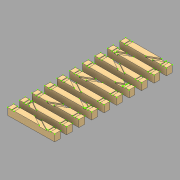
# Autodesk Inventor part: dormentaçãoAmelhor
Saved by Autodesk Inventor 2018 (Build 220112000, 112)
## iProperties
Created: 2019-03-28
Part Number: dormentaçãoAmelhor
Material: Laminated Veneer Lumber
Document SubType Name: Modeling
Designer: Ifes-Vale
Density: 0.51 g/cm^3
Appearance: Plywood - New
Author: Ifes-Vale
Autodesk Inventor part; units mm, degrees
ref_plane "YZ Plane" through (0, 0, 0) normal (1, 0, 0) x (0, 1, 0)
ref_plane "XZ Plane" through (0, 0, 0) normal (0, 1, 0) x (-1, 0, 0)
ref_plane "XY Plane" through (0, 0, 0) normal (0, 0, 1) x (1, 0, 0)
sketch "Sketch2" plane through (0, 0, 0) normal (0, 0, 1) x (1, 0, 0)
  point P0 (264.349385, -5730.127221)
  point P1 (559.859477, -5726.313145)
  point P2 (-178.915755, -5487.873693)
  point P3 (116.594338, -5484.059617)
  point P4 (-663.737, -5225.006632)
  point P5 (-363.609562, -5221.346521)
  point P6 (-677.589036, -4977.200919)
  point P7 (-793.022666, -4978.608654)
  point P8 (-151.211683, -4681.410236)
  point P9 (-451.339121, -4685.099849)
  point P10 (296.670801, -4427.929556)
  point P11 (-3.456637, -4431.61917)
  point P12 (546.007442, -4122.594488)
  point P13 (582.946203, -4121.993825)
  point P14 (144.298409, -3881.152056)
  point P15 (435.191157, -3876.421835)
  point P16 (-372.844253, -3598.273291)
  point P17 (-77.33416, -3595.548009)
  point P18 (-806.874702, -3354.301407)
  point P19 (-525.216644, -3351.703873)
  point P20 (-400.548324, -3051.488745)
  point P21 (-700.675762, -3054.906687)
  point P22 (47.33416, -2798.413483)
  point P23 (-252.793278, -2801.831425)
  point P24 (582.946203, -2497.963106)
  point P25 (287.436111, -2499.067902)
  point P26 (384.40036, -2250.730749)
  point P27 (-141.976993, -1963.360803)
  point P28 (158.150445, -1962.423657)
  point P29 (-594.476822, -1716.799089)
  point P30 (-294.349385, -1715.861943)
  point P31 (-696.058417, -1417.102323)
  point P32 (-252.793278, -1168.024169)
  point P33 (-548.30337, -1168.759844)
  point P34 (264.349385, -877.258052)
  point P35 (-31.160708, -878.112001)
  point P36 (412.104431, -628.856435)
  point P37 (-903.838951, -5745.204739)
  point P38 (-788.405321, -5743.714866)
  point P39 (633.737, -5725.359626)
  point P40 (749.17063, -5723.869752)
  point P41 (-908.456296, -5497.289692)
  point P42 (-793.022666, -5495.799819)
  point P43 (629.119655, -5477.444579)
  point P44 (744.553285, -5475.954706)
  point P45 (-908.456296, -5227.99103)
  point P46 (-793.022666, -5226.583295)
  point P47 (629.119655, -5209.24)
  point P48 (744.553285, -5207.832265)
  point P49 (-913.073641, -4980.072698)
  point P50 (-797.640011, -4978.664963)
  point P51 (629.119655, -4961.265358)
  point P52 (739.93594, -4959.913933)
  point P53 (-913.073641, -4690.776177)
  point P54 (-797.640011, -4689.357095)
  point P55 (624.50231, -4671.874005)
  point P56 (739.93594, -4670.454923)
  point P57 (-917.690986, -4442.858299)
  point P58 (-802.257356, -4441.439217)
  point P59 (624.50231, -4423.899364)
  point P60 (739.93594, -4422.480282)
  point P61 (-917.690986, -4146.395758)
  point P62 (-802.257356, -4144.518686)
  point P63 (624.50231, -4121.318079)
  point P64 (735.318595, -4119.51609)
  point P65 (-917.690986, -3898.421116)
  point P66 (-806.874702, -3896.619127)
  point P67 (619.884965, -3873.41852)
  point P68 (735.318595, -3871.541448)
  point P69 (-922.308332, -3603.340612)
  point P70 (-806.874702, -3602.276049)
  point P71 (619.884965, -3589.118046)
  point P72 (735.318595, -3588.053483)
  point P73 (-922.308332, -3355.365971)
  point P74 (-811.492047, -3354.34399)
  point P75 (615.26762, -3341.185987)
  point P76 (730.70125, -3340.121424)
  point P77 (-926.925677, -3057.483289)
  point P78 (-811.492047, -3056.168696)
  point P79 (615.26762, -3039.920328)
  point P80 (730.70125, -3038.605735)
  point P81 (-926.925677, -2809.508647)
  point P82 (-816.109392, -2808.246638)
  point P83 (615.26762, -2791.945686)
  point P84 (726.083904, -2790.683677)
  point P85 (-931.543022, -2503.62519)
  point P86 (-816.109392, -2503.193628)
  point P87 (610.650274, -2497.859531)
  point P88 (726.083904, -2497.42797)
  point P89 (-931.543022, -2255.650548)
  point P90 (-820.726737, -2255.236249)
  point P91 (610.650274, -2249.884889)
  point P92 (726.083904, -2249.453328)
  point P93 (-936.160367, -1965.840636)
  point P94 (-820.726737, -1965.480195)
  point P95 (610.650274, -1961.010729)
  point P96 (721.466559, -1960.664706)
  point P97 (-936.160367, -1717.865994)
  point P98 (-820.726737, -1717.505553)
  point P99 (606.032929, -1713.050505)
  point P100 (721.466559, -1712.690064)
  point P101 (-940.777712, -1417.711554)
  point P102 (-825.344082, -1417.424181)
  point P103 (606.032929, -1413.860756)
  point P104 (721.466559, -1413.573383)
  point P105 (-940.777712, -1169.736912)
  point P106 (-825.344082, -1169.449539)
  point P107 (601.415584, -1165.897609)
  point P108 (716.849214, -1165.610236)
  point P109 (-945.395058, -880.753908)
  point P110 (-829.961428, -880.420334)
  point P111 (601.415584, -876.284016)
  point P112 (716.849214, -875.950442)
  point P113 (-945.395058, -632.779266)
  point P114 (-829.961428, -632.445692)
  point P115 (601.415584, -628.309374)
  point P116 (712.231869, -627.989143)
  point P117 (-1074.680723, -5747.409752)
  point P118 (915.395058, -5721.724335)
  point P119 (-1074.680723, -5499.43511)
  point P120 (915.395058, -5473.749693)
  point P121 (-1083.915413, -5230.130788)
  point P122 (906.160367, -5205.861436)
  point P123 (-1083.915413, -4982.156146)
  point P124 (906.160367, -4957.886794)
  point P125 (-1088.532759, -4692.933182)
  point P126 (901.543022, -4668.468209)
  point P127 (-1088.532759, -4444.95854)
  point P128 (901.543022, -4420.493567)
  point P129 (-1093.150104, -4149.248907)
  point P130 (896.925677, -4116.888189)
  point P131 (-1093.150104, -3901.274265)
  point P132 (896.925677, -3868.913548)
  point P133 (-1097.767449, -3604.958749)
  point P134 (892.308332, -3586.605677)
  point P135 (-1097.767449, -3356.984107)
  point P136 (892.308332, -3338.631035)
  point P137 (-1107.002139, -3059.534054)
  point P138 (883.073641, -3036.870472)
  point P139 (-1107.002139, -2811.559412)
  point P140 (883.073641, -2788.895831)
  point P141 (-1111.619485, -2504.298425)
  point P142 (878.456296, -2496.858309)
  point P143 (-1111.619485, -2256.323783)
  point P144 (878.456296, -2248.883667)
  point P145 (-1116.23683, -1966.402923)
  point P146 (873.838951, -1960.188924)
  point P147 (-1116.23683, -1718.428282)
  point P148 (873.838951, -1712.214283)
  point P149 (-1125.47152, -1418.171351)
  point P150 (864.60426, -1413.21704)
  point P151 (-1125.47152, -1170.196709)
  point P152 (864.60426, -1165.242399)
  point P153 (-1130.088865, -881.287626)
  point P154 (859.986915, -875.53681)
  point P155 (-1130.088865, -633.312984)
  point P156 (859.986915, -627.562168)
  point P157 (-793.022666, -5042.665596)
  point P158 (-793.022666, -5153.141257)
  point P159 (-793.022666, -5042.665596)
  point P160 (-793.022666, -5153.141257)
  point P161 (619.884965, -4081.420913)
  point P162 (619.884965, -3976.239705)
  point P163 (619.884965, -4081.420913)
  point P164 (619.884965, -3976.239705)
  point P165 (610.650274, -2481.180008)
  point P166 (610.650274, -2315.863581)
  point P167 (610.650274, -2374.7426)
  point P168 (610.650274, -2481.180008)
  point P169 (610.650274, -2315.863581)
  point P170 (610.650274, -2374.7426)
  point P171 (-825.344082, -1325.870433)
  point P172 (-825.344082, -1325.870433)
  point P173 (596.798239, -689.947889)
  point P174 (596.798239, -689.947889)
sketch "Sketch3" plane through (0, 0, 0) normal (0, 0, 1) x (1, 0, 0)
  line L0 (-1130.088865, -633.312984) -> (-1130.088865, -881.287626)
  line L1 (-1130.088865, -881.287626) -> (859.986915, -875.53681)
  line L2 (859.986915, -875.53681) -> (859.986915, -627.562168)
  line L3 (859.986915, -627.562168) -> (-1130.088865, -633.312984)
  line L4 (864.60426, -1165.242399) -> (-1125.47152, -1170.196709)
  line L5 (-1125.47152, -1170.196709) -> (-1125.47152, -1418.171351)
  line L6 (-1125.47152, -1418.171351) -> (864.60426, -1413.21704)
  line L7 (864.60426, -1413.21704) -> (864.60426, -1165.242399)
  line L8 (873.838951, -1712.214283) -> (-1116.23683, -1718.428282)
  line L9 (-1116.23683, -1718.428282) -> (-1116.23683, -1966.402923)
  line L10 (-1116.23683, -1966.402923) -> (873.838951, -1960.188924)
  line L11 (873.838951, -1960.188924) -> (873.838951, -1712.214283)
  line L12 (878.456296, -2248.883667) -> (878.456296, -2496.858309)
  line L13 (878.456296, -2496.858309) -> (-1111.619485, -2504.298425)
  line L14 (-1111.619485, -2504.298425) -> (-1111.619485, -2256.323783)
  line L15 (-1111.619485, -2256.323783) -> (878.456296, -2248.883667)
  line L16 (883.073641, -2788.895831) -> (-1107.002139, -2811.559412)
  line L17 (-1107.002139, -2811.559412) -> (-1107.002139, -3059.534054)
  line L18 (-1107.002139, -3059.534054) -> (883.073641, -3036.870472)
  line L19 (883.073641, -3036.870472) -> (883.073641, -2788.895831)
  line L20 (892.308332, -3338.631035) -> (892.308332, -3586.605677)
  line L21 (892.308332, -3586.605677) -> (-1097.767449, -3604.958749)
  line L22 (-1097.767449, -3604.958749) -> (-1097.767449, -3356.984107)
  line L23 (-1097.767449, -3356.984107) -> (892.308332, -3338.631035)
  line L24 (896.925677, -3868.913548) -> (-1093.150104, -3901.274265)
  line L25 (-1093.150104, -3901.274265) -> (-1093.150104, -4149.248907)
  line L26 (-1093.150104, -4149.248907) -> (896.925677, -4116.888189)
  line L27 (896.925677, -4116.888189) -> (896.925677, -3868.913548)
  line L28 (901.543022, -4420.493567) -> (-1088.532759, -4444.95854)
  line L29 (-1088.532759, -4444.95854) -> (-1088.532759, -4692.933182)
  line L30 (-1088.532759, -4692.933182) -> (901.543022, -4668.468209)
  line L31 (901.543022, -4420.493567) -> (901.543022, -4668.468209)
  line L32 (906.160367, -4957.886794) -> (-1083.915413, -4982.156146)
  line L33 (-1083.915413, -4982.156146) -> (-1083.915413, -5230.130788)
  line L34 (-1083.915413, -5230.130788) -> (906.160367, -5205.861436)
  line L35 (906.160367, -5205.861436) -> (906.160367, -4957.886794)
  line L36 (-1074.680723, -5499.43511) -> (-1074.680723, -5747.409752)
  line L37 (-1074.680723, -5747.409752) -> (915.395058, -5721.724335)
  line L38 (915.395058, -5721.724335) -> (915.395058, -5473.749693)
  line L39 (915.395058, -5473.749693) -> (-1074.680723, -5499.43511)
  point P0 (0, 0)
  constraints: 80 end point, 7 parallel, 6 vertical
extrude "Extrusion1" add sketch "Sketch3" against normal blind 300
sketch "Sketch4" plane through (0, 0, 0) normal (0, 0, 1) x (1, 0, 0)
  line L0 (-903.838951, -5745.204739) -> (-788.405321, -5743.714866)
  line L1 (915.395058, -5721.724335) -> (-1074.680723, -5747.409752)
  line L2 (-793.022666, -5495.799819) -> (-908.456296, -5497.289692)
  line L3 (-908.456296, -5497.289692) -> (-903.838951, -5745.204739)
  line L4 (915.395058, -5473.749693) -> (-1074.680723, -5499.43511)
  line L5 (-788.405321, -5743.714866) -> (-793.022666, -5495.799819)
  line L6 (-793.022666, -5226.583295) -> (-797.640011, -4978.664963)
  line L7 (-797.640011, -4978.664963) -> (-913.073641, -4980.072698)
  line L8 (-1083.915413, -4982.156146) -> (906.160367, -4957.886794)
  line L9 (-908.456296, -5227.99103) -> (-913.073641, -4980.072698)
  line L10 (-793.022666, -5226.583295) -> (-908.456296, -5227.99103)
  line L11 (906.160367, -5205.861436) -> (-1083.915413, -5230.130788)
  line L12 (-797.640011, -4689.357095) -> (-913.073641, -4690.776177)
  line L13 (901.543022, -4668.468209) -> (-1088.532759, -4692.933182)
  line L14 (-913.073641, -4690.776177) -> (-917.690986, -4442.858299)
  line L15 (-917.690986, -4442.858299) -> (-802.257356, -4441.439217)
  line L16 (-1088.532759, -4444.95854) -> (901.543022, -4420.493567)
  line L17 (-802.257356, -4441.439217) -> (-797.640011, -4689.357095)
  line L18 (-917.690986, -4146.395758) -> (-802.257356, -4144.518686)
  line L19 (896.925677, -4116.888189) -> (-1093.150104, -4149.248907)
  line L20 (-802.257356, -4144.518686) -> (-806.874702, -3896.619127)
  line L21 (-806.874702, -3896.619127) -> (-917.690986, -3898.421116)
  line L22 (-1093.150104, -3901.274265) -> (896.925677, -3868.913548)
  line L23 (-917.690986, -4146.395758) -> (-917.690986, -3898.421116)
  line L24 (-922.308332, -3603.340612) -> (-806.874702, -3602.276049)
  line L25 (-806.874702, -3602.276049) -> (-806.874702, -3354.301407)
  line L26 (-806.874702, -3354.301407) -> (-922.308332, -3355.365971)
  line L27 (892.308332, -3338.631035) -> (-1097.767449, -3356.984107)
  line L28 (-922.308332, -3355.365971) -> (-922.308332, -3603.340612)
  line L29 (-926.925677, -3057.483289) -> (-926.925677, -2809.508647)
  line L30 (-926.925677, -2809.508647) -> (-816.109392, -2808.246638)
  line L31 (-1107.002139, -2811.559412) -> (883.073641, -2788.895831)
  line L32 (883.073641, -3036.870472) -> (-1107.002139, -3059.534054)
  line L33 (-811.492047, -3056.168696) -> (-816.109392, -2808.246638)
  line L34 (-926.925677, -3057.483289) -> (-811.492047, -3056.168696)
  line L35 (-931.543022, -2255.650548) -> (-820.726737, -2255.236249)
  line L36 (-1111.619485, -2256.323783) -> (878.456296, -2248.883667)
  line L37 (-816.109392, -2503.193628) -> (-931.543022, -2503.62519)
  line L38 (878.456296, -2496.858309) -> (-1111.619485, -2504.298425)
  line L39 (-931.543022, -2503.62519) -> (-931.543022, -2255.650548)
  line L40 (-820.726737, -2255.236249) -> (-816.109392, -2503.193628)
  line L41 (-820.726737, -1965.480195) -> (-820.726737, -1717.505553)
  line L42 (-820.726737, -1717.505553) -> (-936.160367, -1717.865994)
  line L43 (-1116.23683, -1718.428282) -> (873.838951, -1712.214283)
  line L44 (-820.726737, -1965.480195) -> (-936.160367, -1965.840636)
  line L45 (873.838951, -1960.188924) -> (-1116.23683, -1966.402923)
  line L46 (-936.160367, -1965.840636) -> (-936.160367, -1717.865994)
  line L47 (-825.344082, -1417.424181) -> (-940.777712, -1417.711554)
  line L48 (-940.777712, -1417.711554) -> (-940.777712, -1417.711554)
  line L49 (-940.777712, -1169.736912) -> (-825.344082, -1169.449539)
  line L50 (-825.344082, -1169.449539) -> (-825.344082, -1417.424181)
  line L51 (-940.777712, -1417.711554) -> (-940.777712, -1169.736912)
  line L52 (-945.395058, -880.753908) -> (-945.395058, -632.779266)
  line L53 (-945.395058, -632.779266) -> (-829.961428, -632.445692)
  line L54 (-829.961428, -632.445692) -> (-829.961428, -880.420334)
  line L55 (-829.961428, -880.420334) -> (-829.961428, -880.420334)
  line L56 (-945.395058, -880.753908) -> (-829.961428, -880.420334)
  line L57 (859.986915, -875.53681) -> (-1130.088865, -881.287626)
  point P0 (0, 0)
  constraints: 84 end point, 15 collinear, 3 parallel, 3 vertical
extrude "Extrusion2" cut sketch "Sketch4" against normal blind 25
sketch "Sketch5" plane through (0, 0, 0) normal (0, 0, 1) x (1, 0, 0)
  line L0 (749.17063, -5723.869752) -> (633.737, -5725.359626)
  line L1 (633.737, -5725.359626) -> (629.119655, -5477.444579)
  line L2 (629.119655, -5477.444579) -> (744.553285, -5475.954706)
  line L3 (-1074.680723, -5499.43511) -> (915.395058, -5473.749693)
  line L4 (915.395058, -5721.724335) -> (-1074.680723, -5747.409752)
  line L5 (744.553285, -5475.954706) -> (749.17063, -5723.869752)
  line L6 (744.553285, -5207.832265) -> (629.119655, -5209.24)
  line L7 (906.160367, -5205.861436) -> (-1083.915413, -5230.130788)
  line L8 (629.119655, -5209.24) -> (629.119655, -4961.265358)
  line L9 (629.119655, -4961.265358) -> (739.93594, -4959.913933)
  line L10 (-1083.915413, -4982.156146) -> (906.160367, -4957.886794)
  line L11 (739.93594, -4959.913933) -> (744.553285, -5207.832265)
  line L12 (739.93594, -4670.454923) -> (624.50231, -4671.874005)
  line L13 (624.50231, -4671.874005) -> (624.50231, -4671.874005)
  line L14 (624.50231, -4671.874005) -> (624.50231, -4423.899364)
  line L15 (624.50231, -4423.899364) -> (739.93594, -4422.480282)
  line L16 (739.93594, -4422.480282) -> (739.93594, -4670.454923)
  line L17 (624.50231, -4121.318079) -> (735.318595, -4119.51609)
  line L18 (735.318595, -4119.51609) -> (735.318595, -4119.51609)
  line L19 (735.318595, -4119.51609) -> (735.318595, -3871.541448)
  line L20 (735.318595, -3871.541448) -> (619.884965, -3873.41852)
  line L21 (-1093.150104, -3901.274265) -> (896.925677, -3868.913548)
  line L22 (619.884965, -3873.41852) -> (624.50231, -4121.318079)
  line L23 (619.884965, -3589.118046) -> (735.318595, -3588.053483)
  line L24 (892.308332, -3586.605677) -> (-1097.767449, -3604.958749)
  line L25 (735.318595, -3588.053483) -> (730.70125, -3340.121424)
  line L26 (730.70125, -3340.121424) -> (615.26762, -3341.185987)
  line L27 (-1097.767449, -3356.984107) -> (892.308332, -3338.631035)
  line L28 (615.26762, -3341.185987) -> (619.884965, -3589.118046)
  line L29 (615.26762, -3039.920328) -> (730.70125, -3038.605735)
  line L30 (883.073641, -3036.870472) -> (-1107.002139, -3059.534054)
  line L31 (730.70125, -3038.605735) -> (726.083904, -2790.683677)
  line L32 (615.26762, -2791.945686) -> (726.083904, -2790.683677)
  line L33 (-1107.002139, -2811.559412) -> (883.073641, -2788.895831)
  line L34 (615.26762, -2791.945686) -> (615.26762, -3039.920328)
  line L35 (726.083904, -2497.42797) -> (610.650274, -2497.859531)
  line L36 (610.650274, -2497.859531) -> (610.650274, -2249.884889)
  line L37 (610.650274, -2249.884889) -> (726.083904, -2249.453328)
  line L38 (726.083904, -2249.453328) -> (726.083904, -2249.453328)
  line L39 (878.456296, -2496.858309) -> (-1111.619485, -2504.298425)
  line L40 (726.083904, -2497.42797) -> (726.083904, -2249.453328)
  line L41 (721.466559, -1960.664706) -> (610.650274, -1961.010729)
  line L42 (873.838951, -1960.188924) -> (-820.726737, -1965.480195)
  line L43 (610.650274, -1961.010729) -> (606.032929, -1713.050505)
  line L44 (606.032929, -1713.050505) -> (721.466559, -1712.690064)
  line L45 (-1116.23683, -1718.428282) -> (873.838951, -1712.214283)
  line L46 (721.466559, -1712.690064) -> (721.466559, -1960.664706)
  line L47 (721.466559, -1413.573383) -> (606.032929, -1413.860756)
  line L48 (864.60426, -1413.21704) -> (-825.344082, -1417.424181)
  line L49 (606.032929, -1413.860756) -> (601.415584, -1165.897609)
  line L50 (601.415584, -1165.897609) -> (716.849214, -1165.610236)
  line L51 (-825.344082, -1169.449539) -> (864.60426, -1165.242399)
  line L52 (716.849214, -1165.610236) -> (721.466559, -1413.573383)
  line L53 (601.415584, -628.309374) -> (712.231869, -627.989143)
  line L54 (859.986915, -627.562168) -> (-829.961428, -632.445692)
  line L55 (712.231869, -627.989143) -> (716.849214, -875.950442)
  line L56 (716.849214, -875.950442) -> (601.415584, -876.284016)
  line L57 (-829.961428, -880.420334) -> (859.986915, -875.53681)
  line L58 (601.415584, -876.284016) -> (601.415584, -628.309374)
  point P0 (0, 0)
  constraints: 86 end point, 13 collinear, 4 vertical, 2 parallel
extrude "Extrusion3" cut sketch "Sketch5" against normal blind 25
sketch "Sketch6" plane through (0, 0, 0) normal (0, 0, 1) x (1, 0, 0)
  line L0 (601.415584, -876.284016) -> (601.415584, -628.309374)
  line L1 (-825.344082, -1169.449539) -> (-825.344082, -1417.424181)
  line L2 (610.650274, -2497.859531) -> (610.650274, -2249.884889)
  line L3 (624.50231, -4121.318079) -> (619.884965, -3873.41852)
  line L4 (-797.640011, -4978.664963) -> (-793.022666, -5226.583295)
  line L5 (559.859477, -5726.313145) -> (116.594338, -5484.059617)
  line L6 (116.594338, -5484.059617) -> (-178.915755, -5487.873693)
  line L7 (629.119655, -5477.444579) -> (-793.022666, -5495.799819)
  line L8 (-178.915755, -5487.873693) -> (264.349385, -5730.127221)
  line L9 (264.349385, -5730.127221) -> (559.859477, -5726.313145)
  line L10 (-788.405321, -5743.714866) -> (633.737, -5725.359626)
  line L11 (-363.609562, -5221.346521) -> (-793.022666, -4978.608654)
  line L12 (-793.022666, -4978.608654) -> (-797.640011, -4978.664963)
  line L13 (-797.640011, -4978.664963) -> (-797.640011, -4978.664963)
  line L14 (-793.022666, -5153.141257) -> (-663.737, -5225.006632)
  line L15 (-663.737, -5225.006632) -> (-363.609562, -5221.346521)
  line L16 (-677.589036, -4977.200919) -> (-793.022666, -5042.665596)
  line L17 (-797.640011, -4978.664963) -> (-677.589036, -4977.200919)
  line L18 (-1083.915413, -4982.156146) -> (906.160367, -4957.886794)
  line L19 (-793.022666, -5042.665596) -> (-796.412305, -5044.583974)
  line L20 (-796.412305, -5044.583974) -> (-797.640011, -4978.664963)
  line L21 (-451.339121, -4685.099849) -> (-151.211683, -4681.410236)
  line L22 (901.543022, -4668.468209) -> (-1088.532759, -4692.933182)
  line L23 (296.670801, -4427.929556) -> (-3.456637, -4431.61917)
  line L24 (-802.257356, -4441.439217) -> (624.50231, -4423.899364)
  line L25 (-151.211683, -4681.410236) -> (296.670801, -4427.929556)
  line L26 (-3.456637, -4431.61917) -> (-451.339121, -4685.099849)
  line L27 (546.007442, -4122.594488) -> (619.884965, -4081.420913)
  line L28 (619.884965, -4081.420913) -> (623.759191, -4081.420913)
  line L29 (735.318595, -4119.51609) -> (624.50231, -4121.318079)
  line L30 (623.759191, -4081.420913) -> (624.50231, -4121.318079)
  line L31 (624.50231, -4121.318079) -> (546.007442, -4122.594488)
  line L32 (582.946203, -4121.993825) -> (144.298409, -3881.152056)
  line L33 (144.298409, -3881.152056) -> (435.191157, -3876.421835)
  line L34 (435.191157, -3876.421835) -> (619.884965, -3976.239705)
  line L35 (619.884965, -3976.239705) -> (624.50231, -4121.318079)
  line L36 (624.50231, -4121.318079) -> (619.884965, -3873.41852)
  line L37 (624.50231, -4121.318079) -> (624.50231, -4121.318079)
  line L38 (624.50231, -4121.318079) -> (582.946203, -4121.993825)
  line L39 (-77.33416, -3595.548009) -> (-372.844253, -3598.273291)
  line L40 (-806.874702, -3354.301407) -> (-806.874702, -3602.276049)
  line L41 (-525.216644, -3351.703873) -> (-806.874702, -3354.301407)
  line L42 (-806.874702, -3354.301407) -> (-806.874702, -3358.905694)
  line L43 (-806.874702, -3361.970726) -> (-372.844253, -3598.273291)
  line L44 (-77.33416, -3595.548009) -> (-525.216644, -3351.703873)
  line L45 (-700.675762, -3054.906687) -> (-400.548324, -3051.488745)
  line L46 (615.26762, -3039.920328) -> (-811.492047, -3056.168696)
  line L47 (-252.793278, -2801.831425) -> (47.33416, -2798.413483)
  line L48 (47.33416, -2798.413483) -> (-400.548324, -3051.488745)
  line L49 (-252.793278, -2801.831425) -> (-700.675762, -3054.906687)
  line L50 (582.946203, -2497.963106) -> (287.436111, -2499.067902)
  line L51 (-816.109392, -2503.193628) -> (610.650274, -2497.859531)
  line L52 (610.650274, -2315.863581) -> (287.436111, -2499.067902)
  line L53 (610.650274, -2315.863581) -> (610.650274, -2481.180008)
  line L54 (610.650274, -2481.180008) -> (582.946203, -2497.963106)
  line L55 (384.40036, -2250.730749) -> (610.650274, -2374.7426)
  line L56 (610.650274, -2374.7426) -> (610.650274, -2249.884889)
  line L57 (610.650274, -2249.884889) -> (384.40036, -2250.730749)
  line L58 (-1111.619485, -2256.323783) -> (878.456296, -2248.883667)
  line L59 (158.150445, -1962.423657) -> (-141.976993, -1963.360803)
  line L60 (610.650274, -1961.010729) -> (-820.726737, -1965.480195)
  line L61 (-594.476822, -1716.799089) -> (-294.349385, -1715.861943)
  line L62 (-820.726737, -1717.505553) -> (606.032929, -1713.050505)
  line L63 (158.150445, -1962.423657) -> (-294.349385, -1715.861943)
  line L64 (-141.976993, -1963.360803) -> (-594.476822, -1716.799089)
  line L65 (-696.058417, -1417.102323) -> (-252.793278, -1168.024169)
  line L66 (-252.793278, -1168.024169) -> (-548.30337, -1168.759844)
  line L67 (-825.344082, -1169.449539) -> (601.415584, -1165.897609)
  line L68 (-548.30337, -1168.759844) -> (-825.344082, -1325.870433)
  line L69 (-825.344082, -1325.870433) -> (-825.344082, -1417.424181)
  line L70 (606.032929, -1413.860756) -> (-825.344082, -1417.424181)
  line L71 (-696.058417, -1417.102323) -> (-825.344082, -1417.424181)
  line L72 (-31.160708, -878.112001) -> (264.349385, -877.258052)
  line L73 (264.349385, -877.258052) -> (596.798239, -689.947889)
  line L74 (596.798239, -689.947889) -> (601.415584, -689.947889)
  line L75 (601.415584, -689.947889) -> (601.415584, -628.309374)
  line L76 (601.415584, -628.309374) -> (412.104431, -628.856435)
  line L77 (-1130.088865, -633.312984) -> (859.986915, -627.562168)
  line L78 (412.104431, -628.856435) -> (-31.160708, -878.112001)
  line L79 (-796.412305, -5044.583974) -> (-793.022666, -5153.141257)
  point P0 (0, 0)
  point P1 (-811.492047, -3354.34399)
  constraints: 118 end point, 18 collinear, 7 point on line, 6 parallel, 3 perpendicular, 1 horizontal, 2 other
extrude "Extrusion4" cut sketch "Sketch6" against normal blind 50 contours L74 L73 L72 L78 L76 L0 | L68 L66 L65 L70 L1 | L54 L50 L52 L55 L2 | L55 L52 L2 | L52 L55 L57 L2 | L35 L28 L3 | L31 L32 L27 L28 L35 | L31 L27 L32 | L28 L27 L32 L33 L34 L35 | L12 L11 L16 L19 L4 | L19 L16 L11 L15 L14 L79 | L17 L16 L11 | L9 L8 L6 L5 | L26 L23 L25 L21 | L39 L43 L40 L41 L44 | L49 L47 L48 L45 | L59 L64 L61 L63
body "Solid1"
